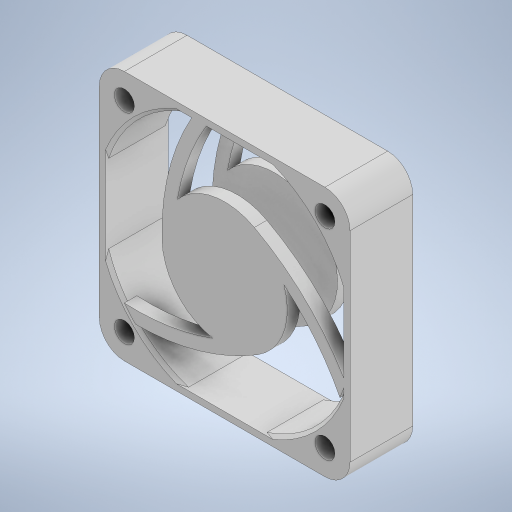
# Autodesk Inventor part: MINI-extruder-fan-DS
Saved by Autodesk Inventor 2023.1 (Build 271208000, 208)
## iProperties
Created: 2022-11-27
Part Number: MINI-extruder-fan-DS
Material: Generic
Document SubType Name: Modeling
Designer: Frank
Density: 1 g/cm^3
Appearance: Default
Author: Frank
Autodesk Inventor part; units mm, degrees
ref_plane "YZ Plane" through (0, 0, 0) normal (1, 0, 0) x (0, 1, 0)
ref_plane "XZ Plane" through (0, 0, 0) normal (0, 1, 0) x (-1, 0, 0)
ref_plane "XY Plane" through (0, 0, 0) normal (0, 0, 1) x (1, 0, 0)
sketch "Sketch1" plane through (0, 0, 0) normal (0, 0, 1) x (1, 0, 0)
  line L0 (-16, -20) -> (16, -20)
  line L1 (20, -16) -> (20, 16)
  line L2 (16, 20) -> (-16, 20)
  line L3 (-20, 16) -> (-20, -16)
  line L4 (-20, -20) -> (20, 20) construction
  line L5 (20, -20) -> (-20, 20) construction
  arc A0 (-16, 20) -> (-20, 16) centre (-16, 16) ccw
  arc A1 (20, 16) -> (16, 20) centre (16, 16) ccw
  arc A2 (16, -20) -> (20, -16) centre (16, -16) ccw
  arc A3 (-20, -16) -> (-16, -20) centre (-16, -16) ccw
  line L6 (-16, 19) -> (16, 19)
  arc A4 (19, 16) -> (16, 19) centre (16, 16) ccw
  line L7 (19, 16) -> (19, -16)
  arc A5 (16, -19) -> (19, -16) centre (16, -16) ccw
  line L8 (16, -19) -> (-16, -19)
  arc A6 (-19, -16) -> (-16, -19) centre (-16, -16) ccw
  line L9 (-19, -16) -> (-19, 16)
  arc A7 (-16, 19) -> (-19, 16) centre (-16, 16) ccw
  arc A8 (-6.245, 19) -> (-19, 6.245) centre (0, 0) ccw
  arc A9 (-19, -6.245) -> (-6.245, -19) centre (0, 0) ccw
  arc A10 (6.245, -19) -> (19, -6.245) centre (0, 0) ccw
  arc A11 (19, 6.245) -> (6.245, 19) centre (0, 0) ccw
  circle A12 centre (0, 0) radius 20 construction
  dimension "d1" = 40
  dimension "d2" = 32
  dimension "d3" = 1
  dimension "d5" = 40
  constraints: 24 point on circle, 20 end point, 16 point on line, 13 centre point, 8 tangent, 7 equal radius, 4 parallel, 3 perpendicular, 2 coincident, 2 midpoint, 1 horizontal, 7 other
  measures "d1" distance between parallel lines of L1 L3
  measures "d2" distance of A1.centre A0.centre
  measures "d3" distance between parallel lines of L2 L6
  measures "d5" diameter of A12
extrude "Extrusion1" add sketch "Sketch1" along normal mid plane 10 contours A3 L3 A0 L2 A1 L1 A2 L0 | L6 A8 L9 A7 | L6 A4 L7 A11 | A9 L8 A6 L9 | L7 A5 L8 A10
sketch "Sketch2" plane through (0, 0, 5) normal (0, 0, 1) x (1, 0, 0)
  arc A0 (19, 6.245) -> (6.245, 19) centre (0, 0) ccw construction
  line L0 (6.245, 19) -> (-6.245, 19) construction
  arc A1 (-6.245, 19) -> (-19, 6.245) centre (0, 0) ccw construction
  line L1 (-19, 6.245) -> (-19, -6.245) construction
  arc A2 (-19, -6.245) -> (-6.245, -19) centre (0, 0) ccw construction
  line L2 (-6.245, -19) -> (6.245, -19) construction
  arc A3 (6.245, -19) -> (19, -6.245) centre (0, 0) ccw construction
  line L3 (19, -6.245) -> (19, 6.245) construction
  line L4 (16, -20) -> (-16, -20) construction
  arc A4 (-20, -16) -> (-16, -20) centre (-16, -16) ccw construction
  line L5 (-20, -16) -> (-20, 16) construction
  arc A5 (-16, 20) -> (-20, 16) centre (-16, 16) ccw construction
  line L6 (-16, 20) -> (16, 20) construction
  arc A6 (20, 16) -> (16, 20) centre (16, 16) ccw construction
  line L7 (20, 16) -> (20, -16) construction
  arc A7 (16, -20) -> (20, -16) centre (16, -16) ccw construction
  circle A8 centre (0, 0) radius 10
  circle A9 centre (0, 0) radius 8
  arc A10 (-5.0388, 19.3549) -> (-9.9953, -0.3059) centre (26.9874, 0.8258) ccw
  arc A11 (-2.3862, 19.8571) -> (-7.9963, -0.2447) centre (26.9874, 0.8258) ccw
  arc A12 (-6.245, 19) -> (-19, 6.245) centre (0, 0) ccw projected
  arc A13 (-2.3862, 19.8571) -> (-5.0388, 19.3549) centre (0, 0) ccw
  arc A14 (-16.0037, -11.9951) -> (4.21, -6.8026) centre (-14.2088, 22.9588) ccw
  arc A15 (-16.0037, -11.9951) -> (-14.2424, -14.0411) centre (0, 0) ccw
  arc A16 (-14.2424, -14.0411) -> (5.2625, -8.5033) centre (-14.2088, 22.9588) ccw
  arc A17 (18.3899, -7.862) -> (3.7862, 7.0473) centre (-12.7785, -23.7846) ccw
  arc A18 (18.3899, -7.862) -> (19.2812, -5.3137) centre (0, 0) ccw
  arc A19 (19.2812, -5.3137) -> (4.7328, 8.8091) centre (-12.7785, -23.7846) ccw
  circle A20 centre (-16, -16) radius 2
  point P0 (-1.9219, -9.8136)
  point P1 (5.2625, -8.5033)
  point P2 (9.4598, 3.2424)
  point P3 (4.7328, 8.8091)
  point P4 (-7.5378, 6.5712)
  dimension "d25" = 20
  dimension "d18" = 2
  dimension "d21" = 360
  dimension "d26" = 35
  dimension "d27" = 4
  constraints: 20 point on circle, 11 coincident, 10 centre point, 1 tangent, 39 other
  measures "d18" radial gap between concentric circles of A10 A11
  measures "d26" radius of A11
  measures "d27" diameter of A20
hole "Hole1" at (-16, 16, 5) at (16, 16, 5) at (16, -16, 5) at (-16, -16, 5) direction (0, 0, -1) diameter 3.2 end through all clearance for "Hex Head Cap Screw ISO 24017" size "M3" standard "ISO"
chamfer "Chamfer1" distance 0.5 angle 45 8 edges at (-14.1421, 14.1421, 5) (-14.1421, 14.1421, -5) (14.1421, 14.1421, 5) (14.1421, 14.1421, -5) (14.1421, -14.1421, 5) (14.1421, -14.1421, -5) (-14.1421, -14.1421, 5) (-14.1421, -14.1421, -5)
extrude "Extrusion2" add sketch "Sketch2" against normal blind 2 contours A8 A14 A9 A17 | A16 A15 A14 A8 | A8 A11 A9 A14 | A17 A9 A11 A8 | A8 A19 A18 A17 | A10 A13 A11 A8 | A9
mirror "Mirror1" about plane through (0, 0, 0) normal (0, 0, 1) of "Extrusion2"
body "Solid1"
